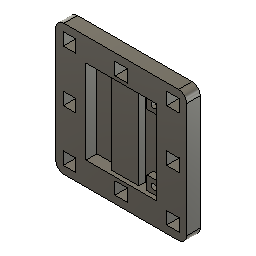
Motor Driver Mount (Autodesk Fusion 360 design; units mm, degrees)
Autodesk Fusion 360 part; units mm, degrees
sketch "Sketch1" plane through (0, 0, 0) normal (0, 0, 1) x (1, 0, 0)
  line L0 (0, 0) -> (-26, 0)
  line L1 (-26, 0) -> (-26, -31)
  line L2 (-26, -31) -> (0, -31)
  line L3 (0, -31) -> (0, 0)
  dimension "d1" = 26
  dimension "d2" = 31
  measures "d1" distance of L0.start
  measures "d2" distance of L0.start
extrude "Extrude1" add sketch "Sketch1" along normal blind 2
sketch "Sketch3" plane through (0, 0, 0) normal (0, 0, -1) x (-1, 0, 0)
  line L0 (0, 0) -> (0, -31)
  line L1 (0, -31) -> (26, -31)
  line L2 (26, -31) -> (26, 0)
  line L3 (26, 0) -> (0, 0)
  line L4 (13, 0) -> (13, -31)
  line L5 (32.05, 3.55) -> (-6.05, 3.55) construction
  line L6 (-6.05, 3.55) -> (-6.05, -34.55) construction
  line L7 (-6.05, -34.55) -> (32.05, -34.55) construction
  line L8 (32.05, -34.55) -> (32.05, 3.55) construction
  line L9 (32.05, 3.55) -> (-6.05, -34.55) construction
  line L10 (-6.05, 3.55) -> (32.05, -34.55) construction
  line L11 (34.3614, 5.8614) -> (29.7386, 5.8614)
  line L12 (29.7386, 5.8614) -> (29.7386, 1.2386)
  line L13 (29.7386, 1.2386) -> (34.3614, 1.2386)
  line L14 (34.3614, 1.2386) -> (34.3614, 5.8614)
  line L15 (34.3614, 5.8614) -> (29.7386, 1.2386) construction
  line L16 (29.7386, 5.8614) -> (34.3614, 1.2386) construction
  line L17 (15.3114, 1.2386) -> (15.3114, 5.8614)
  line L18 (15.3114, 5.8614) -> (10.6886, 5.8614)
  line L19 (10.6886, 5.8614) -> (10.6886, 1.2386)
  line L20 (10.6886, 1.2386) -> (15.3114, 1.2386)
  line L21 (-3.7386, 1.2386) -> (-3.7386, 5.8614)
  line L22 (-3.7386, 5.8614) -> (-8.3614, 5.8614)
  line L23 (-8.3614, 5.8614) -> (-8.3614, 1.2386)
  line L24 (-8.3614, 1.2386) -> (-3.7386, 1.2386)
  line L25 (34.3614, -17.8114) -> (34.3614, -13.1886)
  line L26 (34.3614, -13.1886) -> (29.7386, -13.1886)
  line L27 (29.7386, -13.1886) -> (29.7386, -17.8114)
  line L28 (29.7386, -17.8114) -> (34.3614, -17.8114)
  line L29 (15.3114, -17.8114) -> (15.3114, -13.1886) construction
  line L30 (15.3114, -13.1886) -> (10.6886, -13.1886) construction
  line L31 (10.6886, -13.1886) -> (10.6886, -17.8114) construction
  line L32 (10.6886, -17.8114) -> (15.3114, -17.8114) construction
  line L33 (-3.7386, -17.8114) -> (-3.7386, -13.1886)
  line L34 (-3.7386, -13.1886) -> (-8.3614, -13.1886)
  line L35 (-8.3614, -13.1886) -> (-8.3614, -17.8114)
  line L36 (-8.3614, -17.8114) -> (-3.7386, -17.8114)
  line L37 (34.3614, -36.8614) -> (34.3614, -32.2386)
  line L38 (34.3614, -32.2386) -> (29.7386, -32.2386)
  line L39 (29.7386, -32.2386) -> (29.7386, -36.8614)
  line L40 (29.7386, -36.8614) -> (34.3614, -36.8614)
  line L41 (15.3114, -36.8614) -> (15.3114, -32.2386)
  line L42 (15.3114, -32.2386) -> (10.6886, -32.2386)
  line L43 (10.6886, -32.2386) -> (10.6886, -36.8614)
  line L44 (10.6886, -36.8614) -> (15.3114, -36.8614)
  line L45 (-3.7386, -36.8614) -> (-3.7386, -32.2386)
  line L46 (-3.7386, -32.2386) -> (-8.3614, -32.2386)
  line L47 (-8.3614, -32.2386) -> (-8.3614, -36.8614)
  line L48 (-8.3614, -36.8614) -> (-3.7386, -36.8614)
  line L49 (37.13, 8.63) -> (-11.13, 8.63)
  line L50 (-11.13, 8.63) -> (-11.13, -39.63)
  line L51 (-11.13, -39.63) -> (37.13, -39.63)
  line L52 (37.13, -39.63) -> (37.13, 8.63)
  dimension "d9" = 38.1
  dimension "d10" = 38.1
  dimension "d11" = 4.6228
  dimension "d14" = -38.1
  dimension "d15" = -38.1
  dimension "d16" = 5.08
  dimension "d17" = 5.08
  dimension "d18" = 5.08
  dimension "d19" = 5.08
  measures "d16" distance of L8 L52
  measures "d17" distance of L5 L49
  measures "d18" distance of L7 L51
  measures "d19" distance of L6 L50
extrude "Extrude3" add sketch "Sketch3" against normal blind 5
fillet "Fillet1" radius 3 4 edges at (11.13, -39.63, 2.5) (-37.13, -39.63, 2.5) (11.13, 8.63, 2.5) (-37.13, 8.63, 2.5)
sketch "Sketch4" plane through (0, 0, 2) normal (0, 0, 1) x (1, 0, 0)
  line L0 (0, -31) -> (0, 0)
  line L1 (0, 0) -> (-26, 0)
  line L2 (-26, 0) -> (-26, -31)
  line L3 (-26, -31) -> (0, -31)
  line L4 (-18, 0) -> (-8, 0)
  line L5 (-8, 0) -> (-8, -31)
  line L6 (-8, -31) -> (-18, -31)
  line L7 (-18, -31) -> (-18, 0)
  dimension "d23" = 10
extrude "Extrude4" add sketch "Sketch4" along normal blind 2.5 contours L1 L3 L4 L5 L6 L7
extrude "Extrude5" cut 1 faces at (-8.9614, -16.2705, 0) along direction (0, 0, 1) blind 1
sketch "Sketch5" plane through (0, 0, 2) normal (0, 0, 1) x (1, 0, 0)
  line L0 (-8, 0) -> (-8, -31)
  line L1 (-8, -31) -> (0, -31)
  line L2 (0, -31) -> (0, 0)
  line L3 (0, 0) -> (-8, 0)
  line L4 (-5, -31) -> (0, -31)
  line L5 (0, -31) -> (0, -26)
  line L6 (0, -26) -> (-5, -26)
  line L7 (-5, -26) -> (-5, -31)
  line L8 (-5, 0) -> (0, 0)
  line L9 (0, 0) -> (0, -5)
  line L10 (0, -5) -> (-5, -5)
  line L11 (-5, -5) -> (-5, 0)
  dimension "d28" = 5
extrude "Extrude6" add sketch "Sketch5" along normal blind 2.5 contours L2 L3 L8 L9 L10 L11 | L1 L2 L4 L5 L6 L7
sketch "Sketch6" plane through (0, 0, 4.5) normal (0, 0, 1) x (1, 0, 0)
  line L0 (-5, -5) -> (0, -5)
  line L1 (0, -5) -> (0, 0)
  line L2 (0, 0) -> (-5, 0)
  line L3 (-5, 0) -> (-5, -5)
  line L4 (-2.5, 0) -> (-2.5, -5) construction
  line L5 (0, -26) -> (-5, -26)
  line L6 (0, -31) -> (-5, -31)
  line L7 (-2.5, -26) -> (-2.5, -31) construction
  circle A0 centre (-2.5, -2.5) radius 1
  circle A1 centre (-2.5, -28.5) radius 1
  dimension "d31" = 2
  dimension "d32" = 2
  measures "d31" diameter of A0
  measures "d32" diameter of A1
extrude "Extrude7" cut sketch "Sketch6" against normal blind 2.5 contours A0 | A1
extrude "Extrude8" add 1 faces at (-23.6833, -34.9076, 5) along direction (0, 0, 1) blind 1
